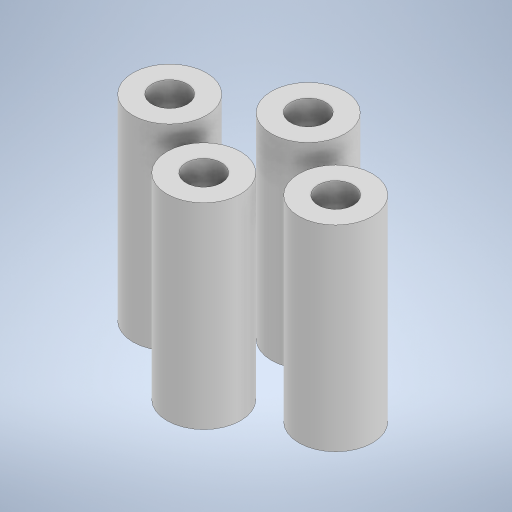
# Autodesk Inventor part: Standoff
Saved by Autodesk Inventor 2023 (Build 270158000, 158)
## iProperties
Created: 2023-07-25
Part Number: Standoff
Material: Generic
Document SubType Name: Modeling
Designer: campstudent
Density: 1 g/cm^3
Appearance: Default
Author: campstudent
Autodesk Inventor part; units mm, degrees
ref_plane "YZ Plane" through (0, 0, 0) normal (1, 0, 0) x (0, 1, 0)
ref_plane "XZ Plane" through (0, 0, 0) normal (0, 1, 0) x (-1, 0, 0)
ref_plane "XY Plane" through (0, 0, 0) normal (0, 0, 1) x (1, 0, 0)
sketch "Sketch1" plane through (0, 0, 0) normal (0, 1, 0) x (-1, 0, 0)
  circle A0 centre (0, 0) radius 1.8
  circle A1 centre (0, 0) radius 3.75
  circle A2 centre (0, -10.6402) radius 1.8
  circle A3 centre (0, -10.6402) radius 3.75
  circle A4 centre (8.6801, -5.2081) radius 1.8
  circle A5 centre (8.6801, -5.2081) radius 3.75
  circle A6 centre (-8.6801, -4.7601) radius 1.8
  circle A7 centre (-8.6801, -4.7601) radius 3.75
  dimension "d0" = 3.6
  dimension "d1" = 7.5
  dimension "d4" = 3.6
  dimension "d5" = 7.5
  dimension "d6" = 3.6
  dimension "d7" = 7.5
  dimension "d8" = 3.6
  dimension "d9" = 7.5
  constraints: 8 centre point, 5 coincident
  measures "d0" diameter of A0
  measures "d1" diameter of A1
  measures "d4" diameter of A2
  measures "d5" diameter of A3
  measures "d6" diameter of A4
  measures "d7" diameter of A5
  measures "d8" diameter of A6
  measures "d9" diameter of A7
extrude "Extrusion1" add sketch "Sketch1" along normal blind 20
body "Solid1"
